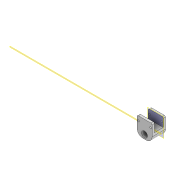
# Autodesk Inventor part: Bearing mount for xrail
Saved by Autodesk Inventor 2020 (Build 240168000, 168)
## iProperties
Created: 2019-12-20
Part Number: Bearing mount for xrail
Material: Generic
Document SubType Name: Modeling
Designer: ball
Density: 1 g/cm^3
Appearance: Default
Author: ball
Autodesk Inventor part; units mm, degrees
ref_plane "YZ Plane" through (0, 0, 0) normal (1, 0, 0) x (0, 1, 0)
ref_plane "XZ Plane" through (0, 0, 0) normal (0, 1, 0) x (-1, 0, 0)
ref_plane "XY Plane" through (0, 0, 0) normal (0, 0, 1) x (1, 0, 0)
ref_plane "Work Plane1" through (0, 0, 0) normal (0, 0, 1) x (1, 0, 0)
sketch "Sketch1" plane through (0, 0, 0) normal (0, 0, 1) x (1, 0, 0)
  line L0 (-9.7566, -4.627) -> (-9.7566, 4.627) construction
  line L1 (-9.7566, -9.525) -> (-314.5566, -9.525) construction
  line L2 (-9.7566, 9.525) -> (-314.5566, 9.525) construction
  line L3 (-42.7766, 3) -> (-42.7766, -3) construction
  line L4 (-9.7566, 9.525) -> (-42.7766, 9.525)
  line L5 (-42.7766, 9.525) -> (-42.7766, -9.525)
  line L6 (-9.7566, -9.525) -> (-9.7566, 9.525)
  line L7 (-9.7566, -9.525) -> (-9.7566, -28.575)
  line L8 (-9.7566, -28.575) -> (-42.7766, -28.575)
  line L9 (-42.7766, -28.575) -> (-42.7766, -9.525)
  arc A0 (-38.0982, 0.6213) -> (-38.1469, -0.737) centre (-39.737, 0) ccw construction
  arc A1 (-11.1575, 0.6213) -> (-11.2061, -0.737) centre (-12.7962, 0) ccw construction
  circle A2 centre (-12.7962, 0) radius 1.9304
  circle A3 centre (-39.737, 0) radius 1.9304
  point P0 (0, 0)
  dimension "d1" = 19.05
  dimension "d2" = 3.8608
  dimension "d3" = 3.8608
  constraints: 12 end point, 2 centre point, 2 coincident, 2 parallel, 1 horizontal, 1 perpendicular, 1 point on line
  measures "d1" distance of L7.start L7.end
  measures "d2" diameter of A2
  measures "d3" diameter of A3
extrude "Extrusion1" add sketch "Sketch1" along normal blind 5.08
ref_plane "Work Plane2" through (0, 0, -19.558) normal (0, 0, -1) x (-1, 0, 0)
sketch "Sketch2" plane through (0, 0, -19.558) normal (0, 0, -1) x (-1, 0, 0)
  line L0 (9.7566, -28.575) -> (9.7566, 9.525) projected
  line L1 (42.7766, 9.525) -> (42.7766, -28.575) projected
  line L2 (9.7566, 9.525) -> (42.7766, 9.525)
  line L3 (42.7766, 9.525) -> (42.7766, -28.575)
  line L4 (42.7766, -28.575) -> (9.7566, -28.575)
  line L5 (9.7566, -28.575) -> (9.7566, 9.525)
  circle A0 centre (12.7962, 0) radius 1.9304 projected
  circle A1 centre (12.7962, 0) radius 1.9304
  circle A2 centre (39.6875, 0) radius 1.9304
  point P0 (0, 0)
  dimension "d7" = 3.8608
  dimension "d8" = 3.8608
  dimension "d24" = 38.1
  dimension "d25" = 9.525
  dimension "d26" = 26.8913
  constraints: 8 end point, 2 centre point, 2 parallel, 1 coincident, 1 horizontal, 1 perpendicular
  measures "d7" diameter of A1
  measures "d8" diameter of A2
  measures "d24" distance between parallel lines of L4 L2
  measures "d25" distance from line of A2.centre L2
  measures "d26" distance of A1.centre A2.centre
extrude "Extrusion2" add sketch "Sketch2" along normal blind 5.08
sketch "Sketch3" plane through (0, 0, 0) normal (0, 0, -1) x (-1, 0, 0)
  line L0 (9.7566, 9.525) -> (42.7766, 9.525) construction
  line L1 (9.7566, 9.525) -> (42.7766, 9.525) construction
  line L2 (42.7766, 9.525) -> (42.7766, -9.525) construction
  line L3 (42.7766, -9.525) -> (9.7566, -9.525) construction
  line L4 (9.7566, -9.525) -> (9.7566, 9.525) construction
  line L5 (42.7766, -28.575) -> (9.7566, -28.575) projected
  line L6 (42.7766, -10.033) -> (42.7766, -28.575)
  line L7 (42.7766, -28.575) -> (9.7566, -28.575)
  line L8 (9.7566, -28.575) -> (9.7566, -10.033)
  line L9 (42.7766, 9.525) -> (42.7766, -28.575) projected
  line L10 (42.7766, -10.033) -> (9.7566, -10.033)
  point P0 (0, 0)
  dimension "d11" = 19.05
  constraints: 16 end point, 3 parallel, 1 horizontal, 1 perpendicular
  measures "d11" distance of L1.end L2.end
extrude "Extrusion3" add sketch "Sketch3" along normal up to surface (19.558 mm away)
sketch "Sketch4" plane through (0, 0, -24.638) normal (0, 0, -1) x (-1, 0, 0)
  circle A0 centre (26.2666, -19.304) radius 6.4135
  line L0 (9.7566, -28.575) -> (42.7766, -28.575) projected
  line L1 (42.7766, -28.575) -> (42.7766, 9.525) projected
  line L2 (9.7566, 9.525) -> (9.7566, -28.575) projected
  line L3 (42.7766, -10.033) -> (9.7566, -10.033) construction
  point P0 (0, 0)
  dimension "d15" = 12.827
  dimension "d16" = 9.271
  dimension "d17" = 33.02
  dimension "d18" = 16.51
  dimension "d19" = 18.542
  constraints: 1 centre point
  measures "d15" diameter of A0
  measures "d16" distance from line of L0 A0.centre
  measures "d17" distance between parallel lines of L1 L2
  measures "d18" distance from line of L2 A0.centre
  measures "d19" distance between parallel lines of L0 L3
extrude "Extrusion4" cut sketch "Sketch4" against normal through all
fillet "Fillet1" radius 12.7 2 edges at (-9.7566, -28.575, -9.779) (-42.7766, -28.575, -9.779)
fillet "Fillet2" radius 2.54 4 edges at (-9.7566, 9.525, -22.098) (-9.7566, 9.525, 2.54) (-42.7766, 9.525, -22.098) (-42.7766, 9.525, 2.54)
equation "\"d16\" = 0.5 * d19"
equation "\"d18\" = 0.5 * d17"
body "Solid1"
